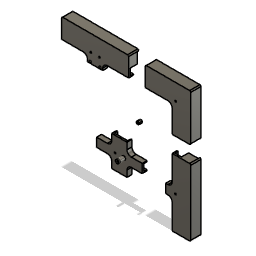
RGBLEDmatrixFrame v11 (Autodesk Fusion 360 design; units mm, degrees)
Autodesk Fusion 360 part; units mm, degrees
sketch "スケッチ1" plane through (0, 0, 0) normal (0, 0, 1) x (1, 0, 0)
  line L0 (60, 60) -> (10, 60)
  line L1 (10, 60) -> (10, 92)
  line L2 (10, 92) -> (90, 92)
  line L3 (90, 92) -> (90, 10)
  line L4 (90, 10) -> (60, 10)
  line L5 (60, 10) -> (60, 60)
  line L6 (-25, 92) -> (-145, 92)
  line L7 (-145, 92) -> (-145, 60)
  line L8 (-145, 60) -> (-24.8, 60)
  line L9 (-25, 60) -> (-25, 92)
  line L10 (-97, 48) -> (-73, 48)
  line L11 (-73, 48) -> (-73, 59.8)
  line L12 (-73, 60) -> (-97, 60)
  line L13 (-97, 59.8) -> (-97, 48)
  line L14 (-85, 59.8) -> (-85, 55)
  circle A0 centre (-77, 64) radius 1.6
  circle A1 centre (-93, 64) radius 1.6
  line L15 (60, 60) -> (48, 60)
  line L16 (60, 48) -> (60, 60)
  line L17 (60, -25) -> (90, -25)
  line L18 (90, -25) -> (90, -145)
  line L19 (90, -145) -> (60, -145)
  line L20 (60, -79) -> (48, -79)
  line L21 (48, -79) -> (48, -91)
  line L22 (48, -91) -> (60, -91)
  circle A2 centre (64, -85) radius 1.6
  line L23 (-80, -68.9376) -> (0, -68.9376)
  line L24 (0, -68.9376) -> (0, -80.9376)
  line L25 (0, -80.9376) -> (-80, -80.9376)
  line L26 (-80, -80.9376) -> (-80, -68.9376)
  line L27 (-40, -60) -> (-40, -90)
  line L28 (-45, -74.9376) -> (-40, -74.9376)
  circle A3 centre (-32, -74.9376) radius 1.6
  circle A4 centre (-48, -74.9376) radius 1.6
  line L29 (-52, -48.9376) -> (-52, -100.9376)
  line L30 (-28, -48.9376) -> (-28, -100.9376)
  line L31 (-52, -48.9376) -> (-28, -48.9376)
  line L32 (-52, -100.9376) -> (-28, -100.9376)
  line L33 (-52.2, -101.1376) -> (-27.8, -101.1376)
  line L34 (-52.2, -48.7376) -> (-27.8, -48.7376)
  line L35 (-80.2, -81.1376) -> (-80.2, -68.7376)
  line L36 (0.2, -68.7376) -> (0.2, -81.1376)
  line L37 (-54.2, -103.1376) -> (-25.8, -103.1376)
  line L38 (-54.2, -46.7376) -> (-25.8, -46.7376)
  line L39 (-82.2, -83.1376) -> (-82.2, -66.7376)
  line L40 (2.2, -66.7376) -> (2.2, -83.1376)
  line L41 (-17.8, -66.7376) -> (2.2, -66.7376)
  line L42 (-25.8, -46.7376) -> (-25.8, -58.7376)
  line L43 (-25.8, -68.7376) -> (-25.8, -68.9376)
  line L44 (-25.8, -80.9376) -> (-25.8, -81.1376)
  line L45 (-25.8, -91.1376) -> (-25.8, -103.1376)
  line L46 (2.2, -83.1376) -> (-17.8, -83.1376)
  line L47 (-54.2, -91.1376) -> (-54.2, -103.1376)
  line L48 (-54.2, -80.9376) -> (-54.2, -81.1376)
  line L49 (-62.2, -83.1376) -> (-82.2, -83.1376)
  line L50 (-54.2, -46.7376) -> (-54.2, -58.7376)
  line L51 (-82.2, -66.7376) -> (-62.2, -66.7376)
  arc A5 (-25.8, -58.7376) -> (-17.8, -66.7376) centre (-17.8, -58.7376) ccw
  arc A6 (-17.8, -83.1376) -> (-25.8, -91.1376) centre (-17.8, -91.1376) ccw
  arc A7 (-54.2, -91.1376) -> (-62.2, -83.1376) centre (-62.2, -91.1376) ccw
  arc A8 (-62.2, -66.7376) -> (-54.2, -58.7376) centre (-62.2, -58.7376) ccw
  line L52 (-52.2, -46.7376) -> (-52.2, -58.5376)
  line L53 (-52.2, -91.3376) -> (-52.2, -103.1376)
  line L54 (-82.2, -68.7376) -> (-62.4, -68.7376)
  line L55 (-17.6, -68.7376) -> (2.2, -68.7376)
  line L56 (-27.8, -46.7376) -> (-27.8, -58.5376)
  line L57 (-27.8, -91.3376) -> (-27.8, -103.1376)
  line L58 (2.2, -81.1376) -> (-17.6, -81.1376)
  line L59 (-62.4, -81.1376) -> (-82.2, -81.1376)
  line L60 (-52.2, -66.7376) -> (-52, -66.7376)
  line L61 (-28, -66.7376) -> (-27.8, -66.7376)
  line L62 (-27.8, -83.1376) -> (-28, -83.1376)
  line L63 (-52, -83.1376) -> (-52.2, -83.1376)
  arc A9 (-27.8, -58.5376) -> (-17.6, -68.7376) centre (-17.6, -58.5376) ccw
  arc A10 (-17.6, -81.1376) -> (-27.8, -91.3376) centre (-17.6, -91.3376) ccw
  arc A11 (-62.4, -68.7376) -> (-52.2, -58.5376) centre (-62.4, -58.5376) ccw
  arc A12 (-52.2, -91.3376) -> (-62.4, -81.1376) centre (-62.4, -91.3376) ccw
  line L64 (-24.8, 59.8) -> (-24.8, 92.2)
  line L65 (-22.8, 92.2) -> (-147.2, 92.2)
  line L66 (-145.2, 92.2) -> (-145.2, 59.8)
  line L67 (-22.8, 57.8) -> (-22.8, 94.2)
  line L68 (-22.8, 94.2) -> (-147.2, 94.2)
  line L69 (-147.2, 94.2) -> (-147.2, 57.8)
  line L70 (-72.8, 45.8) -> (-72.8, 49.6)
  line L71 (-97.2, 49.6) -> (-97.2, 45.8)
  line L72 (-97.2, 47.8) -> (-72.8, 47.8)
  line L73 (-70.8, 45.8) -> (-70.8, 49.8)
  line L74 (-99.2, 49.8) -> (-99.2, 45.8)
  line L75 (-99.2, 45.8) -> (-70.8, 45.8)
  line L76 (-147.2, 59.8) -> (-107.4, 59.8)
  line L77 (-62.6, 59.8) -> (-22.8, 59.8)
  line L78 (-147.2, 57.8) -> (-107.2, 57.8)
  line L79 (-62.8, 57.8) -> (-22.8, 57.8)
  arc A13 (-99.2, 49.8) -> (-107.2, 57.8) centre (-107.2, 49.8) ccw
  arc A14 (-62.8, 57.8) -> (-70.8, 49.8) centre (-62.8, 49.8) ccw
  arc A15 (-97.2, 49.6) -> (-107.4, 59.8) centre (-107.4, 49.6) ccw
  arc A16 (-62.6, 59.8) -> (-72.8, 49.6) centre (-62.6, 49.6) ccw
  line L80 (-147.2, 72) -> (-22.8, 72)
  line L81 (-147.2, 72.2) -> (-22.8, 72.2)
  line L82 (-147.2, 74.2) -> (-22.8, 74.2)
  line L83 (9.8, 72) -> (72, 72)
  line L84 (72, 72) -> (72, 10)
  line L85 (49.6, 59.8) -> (7.8, 59.8)
  line L86 (9.8, 59.8) -> (9.8, 92.2)
  line L87 (7.8, 92.2) -> (90.2, 92.2)
  line L88 (90.2, 92.2) -> (90.2, 7.8)
  line L89 (90.2, 9.8) -> (59.8, 9.8)
  line L90 (59.8, 7.8) -> (59.8, 49.6)
  line L91 (49.8, 57.8) -> (7.8, 57.8)
  line L92 (7.8, 57.8) -> (7.8, 94.2)
  line L93 (7.8, 94.2) -> (92.2, 94.2)
  line L94 (92.2, 94.2) -> (92.2, 7.8)
  line L95 (92.2, 7.8) -> (57.8, 7.8)
  line L96 (57.8, 7.8) -> (57.8, 49.8)
  line L97 (7.8, 72.2) -> (72.2, 72.2)
  line L98 (72.2, 72.2) -> (72.2, 7.8)
  line L99 (7.8, 74.2) -> (74.2, 74.2)
  line L100 (74.2, 74.2) -> (74.2, 7.8)
  arc A17 (57.8, 49.8) -> (49.8, 57.8) centre (49.8, 49.8) ccw
  arc A18 (59.8, 49.6) -> (49.6, 59.8) centre (49.6, 49.6) ccw
  line L101 (72, -25) -> (72, -145)
  line L102 (90.2, -22.8) -> (90.2, -147.2)
  line L103 (90.2, -145.2) -> (59.8, -145.2)
  line L104 (59.8, -24.8) -> (90.2, -24.8)
  line L105 (92.2, -22.8) -> (92.2, -147.2)
  line L106 (92.2, -147.2) -> (57.8, -147.2)
  line L107 (57.8, -22.8) -> (92.2, -22.8)
  line L108 (45.8, -91.2) -> (49.6, -91.2)
  line L109 (49.6, -78.8) -> (45.8, -78.8)
  line L110 (47.8, -78.8) -> (47.8, -91.2)
  line L111 (45.8, -93.2) -> (49.8, -93.2)
  line L112 (49.8, -76.8) -> (45.8, -76.8)
  line L113 (45.8, -76.8) -> (45.8, -93.2)
  line L114 (60, -145) -> (60, -91)
  line L115 (60, -79) -> (60, -25)
  line L116 (59.8, -147.2) -> (59.8, -101.4)
  line L117 (59.8, -68.6) -> (59.8, -22.8)
  line L118 (57.8, -147.2) -> (57.8, -101.2)
  line L119 (57.8, -68.8) -> (57.8, -22.8)
  arc A19 (49.8, -76.8) -> (57.8, -68.8) centre (49.8, -68.8) ccw
  arc A20 (57.8, -101.2) -> (49.8, -93.2) centre (49.8, -101.2) ccw
  arc A21 (49.6, -78.8) -> (59.8, -68.6) centre (49.6, -68.6) ccw
  arc A22 (59.8, -101.4) -> (49.6, -91.2) centre (49.6, -101.4) ccw
  line L120 (72.2, -22.8) -> (72.2, -147.2)
  line L121 (74.2, -22.8) -> (74.2, -147.2)
  circle A23 centre (-32, -74.9376) radius 3.5
  circle A24 centre (-32, -74.9376) radius 2.75
  circle A25 centre (64, 64) radius 1.6
  circle A26 centre (-94, 48.5) radius 2
  circle A27 centre (-76, 48.5) radius 2
  circle A28 centre (0, 0) radius 1.5
  line L122 (2.5, 1.4434) -> (0, 2.8868)
  line L123 (0, 2.8868) -> (-2.5, 1.4434)
  line L124 (-2.5, 1.4434) -> (-2.5, -1.4434)
  line L125 (-2.5, -1.4434) -> (0, -2.8868)
  line L126 (0, -2.8868) -> (2.5, -1.4434)
  line L127 (2.5, -1.4434) -> (2.5, 1.4434)
  dimension "d3" = 50
  dimension "d4" = 50
  dimension "d8" = 120
  dimension "d10" = 12
  dimension "d13" = 3.2
  dimension "d15" = 8
  dimension "d16" = 3.2
  dimension "d18" = 8
  dimension "d19" = 12
  dimension "d20" = 12
  dimension "d22" = 120
  dimension "d23" = 12
  dimension "d27" = 3.2
  dimension "d33" = 60
  dimension "d34" = 80
  dimension "d35" = 12
  dimension "d36" = 40
  dimension "d37" = 6
  dimension "d38" = 3.2
  dimension "d39" = 8
  dimension "d40" = 6
  dimension "d41" = 3.2
  dimension "d42" = 6
  dimension "d43" = 8
  dimension "d44" = 12
  dimension "d45" = 12
  dimension "d46" = 20
  dimension "d47" = 20
  dimension "d52" = 8
  dimension "d53" = 10.2
  dimension "d54" = 10.2
  dimension "d55" = 10.2
  dimension "d56" = 10.2
  dimension "d59" = 12
  dimension "d60" = 12
  dimension "d63" = 8
  dimension "d64" = 8
  dimension "d65" = 10.2
  dimension "d66" = 10.2
  dimension "d67" = 12
  dimension "d68" = -0.2
  dimension "d69" = -2.2
  dimension "d70" = 12
  dimension "d76" = 8
  dimension "d77" = 10.2
  dimension "d80" = 6
  dimension "d81" = 6
  dimension "d82" = 12
  dimension "d84" = -2.2
  dimension "d87" = 8
  dimension "d88" = 8
  dimension "d89" = 10.2
  dimension "d90" = 10.2
  dimension "d104" = 7
  dimension "d107" = 5.5
  dimension "d119" = 3.2
  dimension "d120" = 8
  dimension "d121" = 8
  dimension "d122" = 8
  dimension "d123" = 8
  dimension "d124" = 8
  dimension "d128" = 4
  dimension "d129" = 11.5
  dimension "d130" = 3
  dimension "d134" = 20
  dimension "d135" = 20
  dimension "d137" = 18
  dimension "d139" = 18
  dimension "d140" = 4
  dimension "d141" = 11.5
  dimension "d142" = 3
  dimension "d143" = 3
  dimension "d144" = 2.5
  constraint horizontal L0
  constraint vertical L1
  constraint horizontal L2
  constraint vertical L3
  constraint horizontal L4
  constraint vertical L5
  constraint horizontal L6
  constraint vertical L7
  constraint horizontal L8
  constraint vertical L9
  constraint horizontal L10
  constraint vertical L11
  constraint horizontal L12
  constraint vertical L13
  constraint coincident L8 L12.start
  constraint perpendicular L10 L14
  constraint horizontal L15
  constraint vertical L16
  constraint horizontal L17
  constraint vertical L18
  constraint horizontal L19
  constraint vertical L114
  constraint horizontal L20
  constraint vertical L21
  constraint horizontal L22
  constraint coincident L20.start L114
  constraint horizontal L23
  constraint vertical L24
  constraint horizontal L25
  constraint vertical L26
  constraint perpendicular L25 L27
  constraint coincident L27 L28.end
  constraint perpendicular L27 L28
  constraint perpendicular L25 L29
  constraint perpendicular L25 L30
  constraint perpendicular L30 L31
  constraint perpendicular L30 L32
  constraint coincident L61.end L56
  constraint collinear L41 L51
  constraint coincident L43.start L54
  constraint collinear L42 L43
  constraint coincident L23 L43.end
  constraint coincident L25 L44.start
  constraint collinear L43 L44
  constraint coincident L44.end L58
  constraint collinear L44 L45
  constraint coincident L62.start L56
  constraint collinear L46 L62
  constraint coincident L48.end L58
  constraint collinear L47 L50
  constraint coincident L25 L48.start
  constraint collinear L48 L50
  constraint coincident L63.end L52
  constraint collinear L49 L62
  constraint coincident L60.start L52
  constraint collinear L51 L60
  constraint tangent L42 A5
  constraint tangent L41 A5
  constraint tangent L45 A6
  constraint tangent L46 A6
  constraint equal A5 A6
  constraint tangent L49 A7
  constraint tangent L47 A7
  constraint equal A5 A7
  constraint tangent L51 A8
  constraint tangent L50 A8
  constraint equal A5 A8
  constraint collinear L52 L53
  constraint collinear L54 L55
  constraint collinear L56 L57
  constraint collinear L58 L59
  constraint coincident L29 L60.end
  constraint collinear L60 L61
  constraint coincident L30 L61.start
  constraint coincident L29 L63.start
  constraint collinear L62 L63
  constraint coincident L30 L62.end
  constraint tangent L56 A9
  constraint tangent L55 A9
  constraint tangent L58 A10
  constraint tangent L57 A10
  constraint tangent L52 A11
  constraint tangent L54 A11
  constraint tangent L59 A12
  constraint tangent L53 A12
  constraint coincident L38 L52.start
  constraint coincident L34.start L52
  constraint coincident L38 L56.start
  constraint coincident L34.end L56
  constraint coincident L40 L55.end
  constraint coincident L36.start L55
  constraint coincident L40 L58.start
  constraint coincident L36.end L58
  constraint coincident L37 L57.end
  constraint coincident L33.end L57
  constraint coincident L37 L53.end
  constraint coincident L33.start L53
  constraint coincident L39 L59.end
  constraint coincident L35.start L59
  constraint coincident L39 L54.start
  constraint coincident L35.end L54
  constraint coincident L14.start L76
  constraint coincident L11.end L76
  constraint coincident L69 L65.end
  constraint coincident L66.start L65
  constraint coincident L69 L76.start
  constraint coincident L66.end L76
  constraint coincident L67 L65.start
  constraint coincident L64.end L65
  constraint coincident L64 L8.end
  constraint coincident L9.start L8
  constraint coincident L67 L77.end
  constraint coincident L64.start L76
  constraint coincident L75 L71.end
  constraint coincident L72.start L71
  constraint coincident L75 L70.start
  constraint coincident L72.end L70
  constraint collinear L76 L77
  constraint collinear L78 L79
  constraint tangent L78 A13
  constraint tangent L74 A13
  constraint tangent L73 A14
  constraint tangent L79 A14
  constraint coincident L13.start L76
  constraint tangent L76 A15
  constraint tangent L71 A15
  constraint tangent L70 A16
  constraint tangent L77 A16
  constraint coincident L69 L80.start
  constraint coincident L67 L80.end
  constraint perpendicular L67 L80
  constraint coincident L4 L84.end
  constraint coincident L92 L87.start
  constraint coincident L86.end L87
  constraint coincident L92 L99.start
  constraint coincident L86 L83.start
  constraint coincident L92 L97.start
  constraint coincident L92 L85.end
  constraint coincident L86.start L85
  constraint coincident L95 L88.end
  constraint coincident L89.start L88
  constraint coincident L95 L100.end
  constraint coincident L95 L98.end
  constraint coincident L95 L90.start
  constraint coincident L89.end L90
  constraint tangent L96 A17
  constraint tangent L91 A17
  constraint tangent L85 A18
  constraint tangent L90 A18
  constraint coincident L17 L101.start
  constraint coincident L19 L101.end
  constraint perpendicular L19 L101
  constraint collinear L114 L115
  constraint collinear L116 L117
  constraint collinear L118 L119
  constraint tangent L112 A19
  constraint tangent L119 A19
  constraint tangent L111 A20
  constraint tangent L118 A20
  constraint tangent L117 A21
  constraint tangent L109 A21
  constraint tangent L108 A22
  constraint tangent L116 A22
  constraint coincident L107 L117.end
  constraint coincident L107 L102.start
  constraint coincident L104.end L102
  constraint coincident L106 L102.end
  constraint coincident L103.start L102
  constraint coincident L106 L116.start
  constraint coincident L113 L108.start
  constraint coincident L110.end L108
  constraint coincident L113 L109.end
  constraint coincident L110.start L109
  constraint coincident L107 L120.start
  constraint coincident L107 L121.start
  constraint coincident L106 L120.end
  constraint coincident L106 L121.end
  constraint concentric A3 A23
  constraint concentric A3 A24
  constraint coincident A28.centre origin
  measures "d3" distance of L0.start L0.end
  measures "d4" distance of L0.start L4.end
  measures "d8" distance of L6.start L6.end
  measures "d10" distance of L8 L10
  measures "d13" diameter of A0
  measures "d15" distance of L14 A0.centre
  measures "d16" diameter of A1
  measures "d18" distance of L14 A1.centre
  measures "d19" distance of L0.start L15.end
  measures "d20" distance of L0.start L16.start
  measures "d22" distance of L17.start L19.end
  measures "d23" distance of L20.start L20.end
  measures "d27" diameter of A2
  measures "d33" distance of L17 A2.centre
  measures "d34" distance of L23.start L23.end
  measures "d35" distance of L23.start L25.end
  measures "d36" distance of L24 L27
  measures "d37" distance of L25 L28
  measures "d38" diameter of A3
  measures "d39" distance of L27 A3.centre
  measures "d40" distance of L25 A3.centre
  measures "d41" diameter of A4
  measures "d42" distance of L25 A4.centre
  measures "d43" distance of L27 A4.centre
  measures "d44" distance of L27 L29
  measures "d45" distance of L27 L30
  measures "d46" distance of L23 L31
  measures "d47" distance of L25 L32
  measures "d52" radius of A5
  measures "d53" radius of A9
  measures "d54" radius of A10
  measures "d55" radius of A11
  measures "d56" radius of A12
  measures "d59" distance of L13 L14
  measures "d60" distance of L11 L14
  measures "d63" radius of A13
  measures "d64" radius of A14
  measures "d65" radius of A15
  measures "d66" radius of A16
  measures "d67" distance of L8 L80
  measures "d70" distance of L0 L83
  measures "d76" radius of A17
  measures "d77" radius of A18
  measures "d80" distance of L20 A2.centre
  measures "d81" distance of L22 A2.centre
  measures "d82" distance of L101 L114
  measures "d87" radius of A19
  measures "d88" radius of A20
  measures "d89" radius of A21
  measures "d90" radius of A22
  measures "d104" diameter of A23
  measures "d107" diameter of A24
  measures "d119" diameter of A25
  measures "d120" distance of L83 A25.centre
  measures "d121" distance of L84 A25.centre
  measures "d122" distance of A2.centre L101
  measures "d123" distance of A0.centre L80
  measures "d124" distance of A1.centre L80
  measures "d128" diameter of A26
  measures "d129" distance of L8 A26.centre
  measures "d130" distance of L13 A26.centre
  measures "d134" distance of L2 L83
  measures "d135" distance of L6 L80
  measures "d137" distance of L3 L84
  measures "d139" distance of L18 L101
  measures "d140" diameter of A27
  measures "d141" distance of L12 A27.centre
  measures "d142" distance of L11 A27.centre
  measures "d143" diameter of A28
  measures "d144" distance of A28.centre L127
extrude "押し出し1" add sketch "スケッチ1" against normal blind 3 contours L0 L1 L4 L5 L15 L16 L83 L85 L86 L89 L90 L98 A18 | L0 L1 L4 L5 L15 L16 L83 L84 | L1 L83 L86 L97 | L1 L4 L83 L84 L97 L98 | L1 L86 L97 L99 | L1 L4 L97 L98 L99 L100 | L85 L86 L92 L97 | L4 L89 L98 L100 | L1 L2 L3 L4 L86 L87 L88 L89 L99 L100 | L1 L2 L3 L4 L99 L100 | L86 L92 L97 L99 | L85 L90 L91 L92 L95 L96 A17 A18 | L89 L90 L95 L98 | L89 L95 L98 L100 | L86 L87 L92 L99 | L88 L89 L95 L100 | L87 L88 L92 L93 L94 L95 | L6 L7 L9 L82 | L6 L7 L9 L64 L65 L66 L82 | L9 L64 L81 L82 | L7 L9 L81 L82 | L7 L66 L81 L82 | L9 L64 L80 L81 | L7 L9 L80 L81 | L64 L67 L81 L82 | L64 L65 L67 L82 | L7 L66 L80 L81 | L65 L66 L69 L82 | L66 L69 L81 L82 | L8 L9 L64 L80 | L7 L8 L9 L12 L80 | L64 L67 L80 L81 | L65 L67 L68 L69 | L7 L8 L10 L12 L64 L66 L70 L71 L72 L76 L77 A15 A16 L80 A26 A27 | L66 L69 L80 L81 | L64 L67 L77 L80 | L66 L69 L76 L80 | L69 L71 L74 L75 L76 L78 A13 A15 | L67 L70 L73 L75 L77 L79 A14 A16 | L70 L71 L72 L75 A26 A27 | L10 L72 A26 A27 | L17 L19 L20 L21 L22 L103 L104 L108 L109 L110 L114 L115 L116 L117 A21 A22 L120 | L17 L19 L20 L21 L22 L101 L114 L115 | L17 L19 L101 L120 | L17 L104 L120 L121 | L17 L19 L120 L121 | L17 L18 L19 L102 L103 L104 L121 | L17 L18 L19 L121 | L104 L107 L120 L121 | L104 L107 L117 L120 | L19 L103 L120 L121 | L102 L104 L107 L121 | L107 L109 L112 L113 L117 L119 A19 A21 | L103 L106 L116 L120 | L103 L106 L120 L121 | L102 L105 L106 L107 | L102 L103 L106 L121 | L106 L108 L111 L113 L116 L118 A20 A22 | L108 L109 L110 L113 | L23 L24 L25 L30 | L23 L25 L27 L30 | L23 L29 L30 L31 | L23 L25 L27 L29 | L25 L29 L30 L32 | L23 L25 L26 L29 | L33 L34 L35 L36 L52 L53 L54 L55 L56 L57 L58 L59 A9 A10 A11 A12 | L37 L39 L47 L49 A7 L53 L59 A12 | L33 L37 L53 L57 | L37 L40 L45 L46 A6 L57 L58 A10 | L35 L39 L54 L59 | L36 L40 L55 L58 | L38 L39 L50 L51 A8 L52 L54 A11 | L38 L40 L41 L42 A5 L55 L56 A9 | L34 L38 L52 L56 | A23 | A24 makes body 1 at (-37.6, -85.4405, 0) makes body 2 at (83.3333, -85, 0) makes body 3 at (54.4718, 84.6298, 0) makes body 4 at (-87.6226, 84.6648, -3)
extrude "押し出し2" add sketch "スケッチ1" against normal blind 6 from surface at -3 contours L1 L83 L86 L97 | L1 L86 L97 L99 | L1 L4 L97 L98 L99 L100 | L4 L89 L98 L100 | L86 L92 L97 L99 | L85 L90 L91 L92 L95 L96 A17 A18 | L89 L95 L98 L100 | L9 L64 L81 L82 | L7 L9 L81 L82 | L7 L66 L81 L82 | L64 L67 L81 L82 | L66 L69 L81 L82 | L69 L71 L74 L75 L76 L78 A13 A15 | L67 L70 L73 L75 L77 L79 A14 A16 | L17 L104 L120 L121 | L17 L19 L120 L121 | L104 L107 L120 L121 | L19 L103 L120 L121 | L107 L109 L112 L113 L117 L119 A19 A21 | L103 L106 L120 L121 | L106 L108 L111 L113 L116 L118 A20 A22 | L37 L39 L47 L49 A7 L53 L59 A12 | L37 L40 L45 L46 A6 L57 L58 A10 | L38 L39 L50 L51 A8 L52 L54 A11 | L38 L40 L41 L42 A5 L55 L56 A9 bodies 2 3 1 4
extrude "押し出し3" add sketch "スケッチ1" against normal blind 13 from surface at -3 contours L1 L2 L3 L4 L86 L87 L88 L89 L99 L100 | L1 L2 L3 L4 L99 L100 | L86 L87 L92 L99 | L88 L89 L95 L100 | L87 L88 L92 L93 L94 L95 | L6 L7 L9 L82 | L6 L7 L9 L64 L65 L66 L82 | L64 L65 L67 L82 | L65 L66 L69 L82 | L65 L67 L68 L69 | L17 L18 L19 L102 L103 L104 L121 | L17 L18 L19 L121 | L102 L104 L107 L121 | L102 L105 L106 L107 | L102 L103 L106 L121 bodies 2 3 4
extrude "押し出し7" add sketch "スケッチ1" against normal blind 7 from surface at -9 contours L1 L86 L97 L99 | L1 L4 L97 L98 L99 L100 | L4 L89 L98 L100 | L86 L92 L97 L99 | L89 L95 L98 L100 | L9 L64 L81 L82 | L7 L9 L81 L82 | L7 L66 L81 L82 | L64 L67 L81 L82 | L66 L69 L81 L82 | L17 L104 L120 L121 | L17 L19 L120 L121 | L104 L107 L120 L121 | L19 L103 L120 L121 | L103 L106 L120 L121 bodies 2 3 4
extrude "押し出し4" add sketch "スケッチ1" against normal blind 3 from surface at -16 contours L87 L88 L92 L93 L94 L95 | L65 L67 L68 L69 | L102 L105 L106 L107 bodies 2 3 4
fillet "フィレット1" radius 2 6 edges at (92.2, -22.8, -9.5) (92.2, -147.2, -9.5) (7.8, 94.2, -9.5) (92.2, 7.8, -9.5) (-22.8, 94.2, -9.5) (-147.2, 94.2, -9.5) on bodies 2 3 4
fillet "フィレット1" radius 2 1 edges at (92.2, 94.2, -9.5) on bodies 2 3 4
extrude "押し出し5" add sketch "スケッチ1" along normal blind 12 separate body contours A23 | A24 makes body 5
extrude "押し出し6" cut sketch "スケッチ1" against normal blind 2.5 from surface at 12 contours A24 bodies 5
extrude "押し出し8" add sketch "スケッチ1" along normal blind 6 separate body contours L122 L123 L124 L125 L126 L127 makes body 6
thread "ねじ1" "ISO Metric profile 3.0 M3x0.5 6H" major diameter 3.086 minor diameter 2.529 pitch 0.5 angle 60 resizes the face on face at (1.4981, -0.0748, 4) on bodies 6
named bodies: "connectorCenter_2_rev2", "connectorLR_2", "connectorCorner_4", "connectorTB_4", "foot_12", "M3_6mm_spacer"
